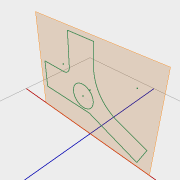
# Autodesk Inventor part: ЛЦМК000002.00.00.00.00.15 Держатель батареи
Saved by Autodesk Inventor 2021.2 (Build 252289000, 289)
## iProperties
Created: 2025-11-04
Part Number: ЛЦМК000002.00.00.00.00.15 Держатель батареи
Material: Типовые
Document SubType Name: Modeling
Designer: Захаров
Density: 1 g/cm^3
Appearance: По умолчанию
Author: Захаров
Autodesk Inventor part; units mm, degrees
ref_plane "YZ Plane" through (0, 0, 0) normal (1, 0, 0) x (0, 1, 0)
ref_plane "XZ Plane" through (0, 0, 0) normal (0, 1, 0) x (-1, 0, 0)
ref_plane "XY Plane" through (0, 0, 0) normal (0, 0, 1) x (1, 0, 0)
ref_plane "РабПлоскость1" through (0, 0, 0) normal (0, 0, 1) x (1, 0, 0)
sketch "Эскиз1" plane through (0, 0, 0) normal (0, 0, 1) x (1, 0, 0)
  line L0 (-1.043, -24.4234) -> (-58.4202, -24.4234) projected
  line L1 (51.5798, -43.5766) -> (-1.043, -24.4234) projected
  line L2 (58.4202, -24.7827) -> (51.5798, -43.5766) projected
  line L3 (32.5787, -15.3772) -> (58.4202, -24.7827) projected
  arc A0 (3.5798, 23.5766) -> (32.5787, -15.3772) centre (44.0796, 23.4555) ccw projected
  line L4 (3.5798, 43.5766) -> (3.5798, 23.5766) projected
  line L5 (-24.4202, 43.5766) -> (3.5798, 43.5766) projected
  line L6 (-24.4202, 12.0766) -> (-24.4202, 43.5766) projected
  arc A1 (-31.4202, 3.5766) -> (-24.4202, 12.0766) centre (-31.8516, 11.0641) ccw projected
  line L7 (-58.4202, 3.5766) -> (-31.4202, 3.5766) projected
  line L8 (-58.4202, -24.4234) -> (-58.4202, 3.5766) projected
  circle A2 centre (-8.4202, -10.3442) radius 12 projected
  circle A3 centre (17.7065, 13.8766) radius 1.65 projected
  circle A4 centre (17.7065, -26.3234) radius 1.65 projected
  circle A5 centre (-32.2935, -26.3234) radius 1.65 projected
  circle A6 centre (-32.2935, 13.8766) radius 1.65 projected
  circle A7 centre (-32.2935, -26.3234) radius 1.65 projected
  circle A8 centre (17.7065, -26.3234) radius 1.65 projected
  circle A9 centre (17.7065, 13.8766) radius 1.65 projected
  circle A10 centre (-32.2935, 13.8766) radius 1.65 projected
  point P0 (0, 0)
ref_plane "РабПлоскость2" through (-8.4202, -10.3442, 4) normal (0, 0, 1) x (1, 0, 0)
sketch "Эскиз2" plane through (-8.4202, -10.3442, 4) normal (0, 0, 1) x (1, 0, 0)
  arc A0 (-17.9957, -19.0702) -> (29.1947, 4.1961) centre (-13.6832, 31.6735) ccw
  circle A1 centre (27.0898, 5.545) radius 2.5
  arc A2 (27.9391, 7.8963) -> (-23.2379, 18.9133) centre (-38.3302, -175.569) ccw
  circle A3 centre (-23.4314, 16.4208) radius 2.5
  arc A4 (-20.2839, -16.5633) -> (-25.7837, 15.5745) centre (-113.4568, -15.9687) ccw
  circle A5 centre (-17.784, -16.5792) radius 2.5
  point P0 (8.4202, 10.3442)
  constraints: 6 centre point, 6 point on circle, 18 other
ref_plane "РабПлоскость3" through (-58.4202, -43.5766, -1.8) normal (0, 0, -1) x (0, 1, 0)
extrude "Выдавливание1" add sketch "Эскиз2" against normal up to surface (5.8 mm away) contours A5 | A1 | A3
ref_plane "РабПлоскость4" through (-22.4202, -24.3442, 2) normal (0, 0, -1) x (0, 1, 0)
extrude "Выдавливание2" add sketch "Эскиз2" along normal blind 2
sketch "Эскиз4" plane through (-8.4202, -10.3442, 4) normal (0, 0, -1) x (-1, 0, 0)
  circle A0 centre (0, 0) radius 14 projected
  circle A1 centre (0, 0) radius 14.5
  arc A2 (-29.1947, 4.1961) -> (17.9957, -19.0702) centre (13.6832, 31.6735) ccw projected
  arc A3 (25.7837, 15.5745) -> (20.2839, -16.5633) centre (113.4568, -15.9687) ccw projected
  arc A4 (23.2379, 18.9133) -> (-27.9391, 7.8963) centre (38.3302, -175.569) ccw projected
  arc A5 (20.2839, -16.5633) -> (17.9957, -19.0702) centre (17.784, -16.5792) ccw projected
  arc A6 (25.7837, 15.5745) -> (20.2839, -16.5633) centre (113.4568, -15.9687) ccw projected
  arc A7 (23.2379, 18.9133) -> (25.7837, 15.5745) centre (23.4314, 16.4208) ccw projected
  arc A8 (23.2379, 18.9133) -> (-27.9391, 7.8963) centre (38.3302, -175.569) ccw projected
  arc A9 (-29.1947, 4.1961) -> (-27.9391, 7.8963) centre (-27.0898, 5.545) ccw projected
  arc A10 (-29.1947, 4.1961) -> (17.9957, -19.0702) centre (13.6832, 31.6735) ccw projected
  point P0 (-8.4202, 10.3442)
  point P1 (17.9957, -19.0702)
  point P2 (20.2839, -16.5633)
  point P3 (25.7837, 15.5745)
  point P4 (23.2379, 18.9133)
  point P5 (-27.9391, 7.8963)
  point P6 (-29.1947, 4.1961)
  dimension "d4" = 0.5
  constraints: 1 centre point
  measures "d4" radial gap between concentric circles of A0 A1
extrude "Выдавливание3" add sketch "Эскиз4" along normal blind 1.25 contours A9 A4 A7 A3 A5 A2
